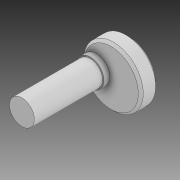
# Autodesk Inventor part: camshaft
Saved by Autodesk Inventor 2020 (Build 240168000, 168)
## iProperties
Created: 2020-11-25
Part Number: camshaft
Material: Generic
Document SubType Name: Modeling
Designer: DDeGo
Density: 1 g/cm^3
Appearance: Default
Author: DDeGo
Autodesk Inventor part; units mm, degrees
ref_plane "YZ Plane" through (0, 0, 0) normal (1, 0, 0) x (0, 1, 0)
ref_plane "XZ Plane" through (0, 0, 0) normal (0, 1, 0) x (-1, 0, 0)
ref_plane "XY Plane" through (0, 0, 0) normal (0, 0, 1) x (1, 0, 0)
sketch "Sketch1" plane through (0, 0, 0) normal (0, 0, 1) x (1, 0, 0)
  circle A0 centre (0, 0) radius 6
  dimension "d0" = 12
  constraints: 1 centre point, 1 coincident
  measures "d0" diameter of A0
extrude "Extrusion1" add sketch "Sketch1" along normal blind 3.5
sketch "Sketch2" plane through (0, 0, 3.5) normal (0, 0, 1) x (1, 0, 0)
  line L0 (0, 0) -> (-3, 0) construction
  circle A0 centre (-3, 0) radius 2.5
  dimension "d3" = 5
  dimension "d4" = 3
  constraints: 2 end point, 1 centre point, 1 coincident, 1 horizontal
  measures "d3" diameter of A0
  measures "d4" distance of L0.start L0.end
extrude "Extrusion2" add sketch "Sketch2" along normal blind 15
sketch "Sketch3" plane through (0, 0, 3.5) normal (0, 0, 1) x (1, 0, 0)
  circle A0 centre (-3, 0) radius 2.5 projected
  circle A1 centre (-3, 0) radius 2.75
  point P0 (0, 0)
  dimension "d7" = 5.5
  constraints: 1 centre point, 1 coincident
  measures "d7" diameter of A1
extrude "Extrusion3" add sketch "Sketch3" along normal blind 1.2
chamfer "Chamfer1" distance 0.5 angle 45 2 edges at (-6, 0, 0) (-6, 0, 3.5)
sketch "Sketch4" plane through (0, 0, 0) normal (0, 0, -1) x (-1, 0, 0)
  circle A0 centre (3, 0) radius 2.5 projected
  point P0 (0, 0)
extrude "Extrusion4" add sketch "Sketch4" along normal blind 3 and the other way blind 1.5
body "Solid1"
